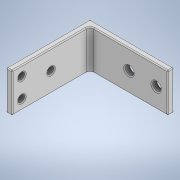
# Autodesk Inventor part: angle_back
Saved by Autodesk Inventor 2022 (Build 260153000, 153)
## iProperties
Created: 2022-03-04
Part Number: angle_back
Material: Generic
Document SubType Name: Modeling
Designer: Frey
Density: 1 g/cm^3
Appearance: Default
Author: Frey
Autodesk Inventor part; units mm, degrees
ref_plane "YZ Plane" through (0, 0, 0) normal (1, 0, 0) x (0, 1, 0)
ref_plane "XZ Plane" through (0, 0, 0) normal (0, 1, 0) x (-1, 0, 0)
ref_plane "XY Plane" through (0, 0, 0) normal (0, 0, 1) x (1, 0, 0)
sketch "Sketch1" plane through (0, 0, 0) normal (0, 0, 1) x (1, 0, 0)
  line L0 (-21.5, 10) -> (21.5, 10)
  line L1 (21.5, 10) -> (21.5, -10)
  line L2 (21.5, -10) -> (-21.5, -10)
  line L3 (-21.5, -10) -> (-21.5, 10)
  line L4 (-21.5, 10) -> (21.5, -10) construction
  line L5 (-21.5, -10) -> (21.5, 10) construction
  point P0 (0, 0)
  point P1 (0, 0)
  point P2 (0, 0)
  dimension "d0" = 20
  dimension "d1" = 43
  constraints: 12 end point, 2 midpoint, 2 parallel, 1 coincident, 1 horizontal, 1 perpendicular
  measures "d0" distance of L0.end L1.end
  measures "d1" distance between parallel lines of L1 L3
extrude "Extrusion1" add sketch "Sketch1" along normal blind 3
sketch "Sketch2" plane through (0, 0, 3) normal (0, 0, 1) x (1, 0, 0)
  line L0 (-21.5, 10) -> (-18.5, 10)
  line L1 (-18.5, 10) -> (-18.5, -10)
  line L2 (-18.5, -10) -> (-21.5, -10)
  line L3 (-21.5, -10) -> (-21.5, 10)
  point P0 (0, 0)
  dimension "d4" = 3
  constraints: 8 end point, 2 horizontal alignment, 2 parallel, 1 horizontal, 1 perpendicular
  measures "d4" distance between parallel lines of L3 L1
extrude "Extrusion2" add sketch "Sketch2" along normal blind 40
sketch "Sketch3" plane through (0, 0, 0) normal (0, 0, -1) x (-1, 0, 0)
  circle A0 centre (-15.5, 0) radius 2.25
  circle A1 centre (-1.5, 0) radius 2.25
  line L0 (18.5, 10) -> (18.5, -10) projected
  point P0 (0, 0)
  dimension "d7" = 4.5
  dimension "d8" = 4.5
  dimension "d9" = 14
  dimension "d10" = 20
  constraints: 2 centre point, 2 horizontal alignment
  measures "d7" diameter of A0
  measures "d8" diameter of A1
  measures "d9" distance of A1.centre A0.centre
  measures "d10" distance from line of A1.centre L0
extrude "Extrusion3" cut sketch "Sketch3" against normal up to surface (3 mm away)
sketch "Sketch4" plane through (-21.5, -10, 0) normal (-1, 0, 0) x (0, 0, 1)
  circle A0 centre (23, 10) radius 1.75
  circle A1 centre (38, 15) radius 1.75
  circle A2 centre (38, 5) radius 1.75
  line L0 (43, 20) -> (43, 0) projected
  line L1 (0, 0) -> (43, 0) projected
  line L2 (0, 20) -> (43, 20) projected
  line L3 (0, 20) -> (0, 0) projected
  point P0 (0, 10)
  point P1 (0, 10)
  dimension "d13" = 3.5
  dimension "d14" = 3.5
  dimension "d15" = 3.5
  dimension "d16" = 15
  dimension "d17" = 5
  dimension "d18" = 10
  dimension "d19" = 20
  dimension "d20" = 5
  constraints: 3 centre point, 1 horizontal alignment, 1 midpoint, 1 vertical alignment
  measures "d13" diameter of A0
  measures "d14" diameter of A1
  measures "d15" diameter of A2
  measures "d16" horizontal distance of A1.centre A0.centre
  measures "d17" distance from line of L0 A1.centre
  measures "d18" distance of A2.centre A1.centre
  measures "d19" distance between parallel lines of L1 L2
  measures "d20" distance from line of L2 A1.centre
extrude "Extrusion4" cut sketch "Sketch4" against normal blind 10 contours A0 | A1 | A2
fillet "Fillet1" radius 2 1 edges at (-18.5, 0, 3)
fillet "Fillet2" radius 0.5 29 edges at (2.5, 10, 3) (-17.9142, 10, 3.5858) (21.5, 10, 1.5) (-18.5, 10, 24) (0, 10, 0) (-20, 10, 43) (-21.5, 10, 21.5) (21.5, 0, 3) (2.5, -10, 3) (3.75, 0, 3) (17.75, 0, 3) (-17.9142, -10, 3.5858) (21.5, -10, 1.5) (21.5, 0, 0) (-18.5, -10, 24) (-18.5, 0, 43) (-18.5, -5, 36.25) (-18.5, 5, 36.25) (-18.5, 0, 21.25) (-21.5, 0, 0) (0, -10, 0) (3.75, 0, 0) (17.75, 0, 0) (-21.5, 0, 43) (-20, -10, 43) (-21.5, -10, 21.5) (-21.5, 5, 36.25) (-21.5, -5, 36.25) (-21.5, 0, 21.25)
body "Solid1"
